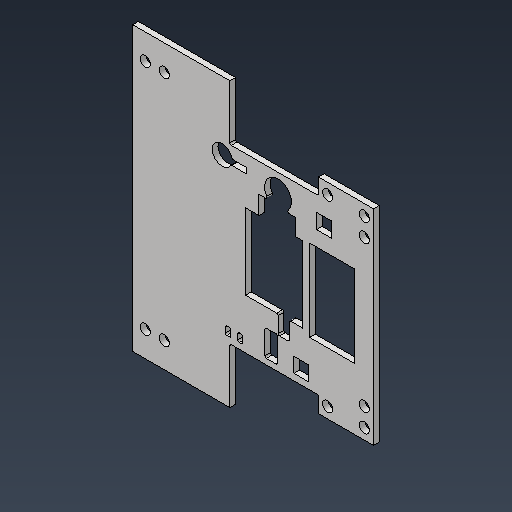
# Autodesk Inventor part: ceil
Saved by Autodesk Inventor 2026.2 (Build 302298010, 298A)
## iProperties
Created: 2026-05-09
Part Number: ceil
Material: Generic
Document SubType Name: Modeling
Designer: szymo
Density: 1 g/cm^3
Appearance: Default
Author: szymo
Autodesk Inventor part; units mm, degrees
ref_plane "YZ Plane" through (0, 0, 0) normal (1, 0, 0) x (0, 1, 0)
ref_plane "XZ Plane" through (0, 0, 0) normal (0, 1, 0) x (-1, 0, 0)
ref_plane "XY Plane" through (0, 0, 0) normal (0, 0, 1) x (1, 0, 0)
sketch "Sketch1" plane through (0, 0, 0) normal (0, 0, 1) x (1, 0, 0)
  circle A0 centre (3.25, 13.15) radius 1.2295 projected
  line L0 (0, 9.3) -> (6.5, 9.3) projected
  line L1 (6.5, 9.3) -> (6.5, 17) projected
  line L2 (0, 17) -> (6.5, 17) projected
  line L3 (0, 9.3) -> (0, 17) projected
  circle A1 centre (3.25, 6.65) radius 1.2295 projected
  line L4 (0, 0) -> (6.5, 0) projected
  line L5 (6.5, 0) -> (6.5, 9.3) projected
  line L6 (6.5, 9.3) -> (0, 9.3) projected
  line L7 (0, 0) -> (0, 9.3) projected
  circle A2 centre (-9.75, 13.15) radius 1.2295 projected
  line L8 (-41.3371, 11.3) -> (-13, 11.3) projected
  line L9 (-41.3371, 9.3) -> (-41.3371, 11.3) projected
  line L10 (-41.3371, 9.3) -> (-6.5, 9.3) projected
  line L11 (-6.5, 9.3) -> (-6.5, 17) projected
  line L12 (-13, 17) -> (-6.5, 17) projected
  line L13 (-13, 11.3) -> (-13, 17) projected
  circle A3 centre (3.25, -51.55) radius 1.2295 projected
  line L14 (0, -47.7) -> (6.5, -47.7) projected
  line L15 (0, -47.7) -> (0, -55.4) projected
  line L16 (6.5, -55.4) -> (0, -55.4) projected
  line L17 (6.5, -47.7) -> (6.5, -55.4) projected
  circle A4 centre (3.25, -45.05) radius 1.2295 projected
  line L18 (0.5983, -42.4) -> (0, -42.4) projected
  line L19 (0, -42.4) -> (0, -47.7) projected
  line L20 (0, -47.7) -> (6.5, -47.7) projected
  line L21 (6.5, -38.4) -> (6.5, -47.7) projected
  line L22 (0.5983, -38.4) -> (6.5, -38.4) projected
  line L23 (0.5983, -38.4) -> (0.5983, -42.4) projected
  circle A5 centre (-9.75, -51.55) radius 1.2295 projected
  line L24 (-41.3371, -47.7) -> (-6.5, -47.7) projected
  line L25 (-41.3371, -47.7) -> (-41.3371, -49.7) projected
  line L26 (-13, -49.7) -> (-41.3371, -49.7) projected
  line L27 (-13, -49.7) -> (-13, -55.4) projected
  line L28 (-6.5, -55.4) -> (-13, -55.4) projected
  line L29 (-6.5, -47.7) -> (-6.5, -55.4) projected
  circle A6 centre (-67.4121, -60.2) radius 1.2295 projected
  circle A7 centre (-74.1621, -60.2) radius 1.2295 projected
  arc A8 (-64.1621, -55.1072) -> (-64.7971, -54.6257) centre (-64.6621, -55.1072) ccw projected
  arc A9 (-65.3371, -54.7) -> (-64.7971, -54.6257) centre (-65.3371, -52.7) ccw projected
  line L30 (-65.3371, -54.7) -> (-78.8451, -54.7) projected
  line L31 (-78.8451, -54.7) -> (-78.8451, -69.2) projected
  line L32 (-59.3371, -69.2) -> (-78.8451, -69.2) projected
  line L33 (-59.3371, -67.7) -> (-59.3371, -69.2) projected
  line L34 (-59.3371, -67.7) -> (-70.1621, -67.7) projected
  line L35 (-70.1621, -67.7) -> (-70.1621, -65.2) projected
  line L36 (-70.1621, -65.2) -> (-67.1621, -65.2) projected
  arc A10 (-67.1621, -65.2) -> (-64.1621, -62.2) centre (-67.1621, -62.2) ccw projected
  line L37 (-64.1621, -62.2) -> (-64.1621, -55.1072) projected
  arc A11 (-64.7971, 16.2257) -> (-64.1621, 16.7072) centre (-64.6621, 16.7072) ccw projected
  line L38 (-64.1621, 16.7072) -> (-64.1621, 23.8) projected
  arc A12 (-64.1621, 23.8) -> (-67.1621, 26.8) centre (-67.1621, 23.8) ccw projected
  line L39 (-67.1621, 26.8) -> (-70.1621, 26.8) projected
  line L40 (-70.1621, 26.8) -> (-70.1621, 29.3) projected
  line L41 (-70.1621, 29.3) -> (-59.3371, 29.3) projected
  line L42 (-59.3371, 29.3) -> (-59.3371, 30.8) projected
  line L43 (-59.3371, 30.8) -> (-78.8451, 30.8) projected
  line L44 (-78.8451, 16.3) -> (-78.8451, 30.8) projected
  line L45 (-65.3371, 16.3) -> (-78.8451, 16.3) projected
  arc A13 (-64.7971, 16.2257) -> (-65.3371, 16.3) centre (-65.3371, 14.3) ccw projected
  circle A14 centre (-67.4121, 21.8) radius 1.2295 projected
  circle A15 centre (-74.1621, 21.8) radius 1.2295 projected
  line L46 (-78.5805, 30.8) -> (-78.5805, -69.2) projected
  line L47 (-44.2868, 25.8) -> (-44.2868, 15.8) projected
  line L48 (-44.2868, -54.2) -> (-44.2868, -64.2) projected
  line L49 (-59.3371, 30.8) -> (-44.2868, 30.8)
  line L50 (-44.2868, 30.8) -> (-44.2868, 11.3)
  line L51 (-44.2868, 11.3) -> (-41.3371, 11.3)
  line L52 (-59.3371, -69.2) -> (-44.2868, -69.2)
  line L53 (-44.2868, -69.2) -> (-44.2868, -64.2)
  line L54 (-44.2868, -54.2) -> (-44.2868, -49.7)
  line L55 (-44.2868, -49.7) -> (-41.3371, -49.7)
  line L56 (-6.5, 17) -> (0, 17)
  line L57 (6.5, 0) -> (6.5, -38.4)
  line L58 (0, -55.4) -> (-6.5, -55.4)
  line L59 (-24.2185, -0.425) -> (-24.4685, -0.675) construction
  line L60 (-24.4685, -0.675) -> (-24.4685, -0.725) construction
  line L61 (-24.4685, -0.725) -> (-24.5685, -0.725) construction
  line L62 (-24.5685, -5.125) -> (-24.5685, -0.725) construction
  line L63 (-24.4685, -5.125) -> (-24.5685, -5.125) construction
  line L64 (-24.4685, -5.125) -> (-24.4685, -5.175) construction
  line L65 (-24.4685, -5.175) -> (-24.2185, -5.425) construction
  line L66 (-24.2185, -5.425) -> (-23.3685, -5.425) construction
  line L67 (-23.3685, -5.925) -> (-23.3685, -5.425) construction
  line L68 (-21.6685, -5.925) -> (-23.3685, -5.925) construction
  line L69 (-21.6685, -5.925) -> (-21.6685, 0.075) construction
  line L70 (-21.6685, 0.075) -> (-23.3685, 0.075) construction
  line L71 (-23.3685, 0.075) -> (-23.3685, -0.425) construction
  line L72 (-24.2185, -0.425) -> (-23.3685, -0.425) construction
  line L73 (-24.2685, -5.225) -> (-23.1685, -5.225) construction
  line L74 (-24.2685, -0.625) -> (-24.2685, -5.225) construction
  line L75 (-24.2685, -0.625) -> (-23.1685, -0.625) construction
  line L76 (-23.1685, -0.625) -> (-23.1685, -0.375) construction
  line L77 (-22.5685, -0.375) -> (-23.1685, -0.375) construction
  line L78 (-22.5685, -0.375) -> (-22.5685, -0.625) construction
  line L79 (-22.5685, -0.625) -> (-21.9685, -0.625) construction
  line L80 (-21.9685, -5.225) -> (-21.9685, -0.625) construction
  line L81 (-22.5685, -5.225) -> (-21.9685, -5.225) construction
  line L82 (-22.5685, -5.475) -> (-22.5685, -5.225) construction
  line L83 (-22.5685, -5.475) -> (-23.1685, -5.475) construction
  line L84 (-23.1685, -5.225) -> (-23.1685, -5.475) construction
  line L85 (-30.9685, -4.8) -> (-30.7185, -4.55) construction
  line L86 (-30.7185, -4.55) -> (-30.7185, -4.5) construction
  line L87 (-30.7185, -4.5) -> (-30.6185, -4.5) construction
  line L88 (-30.6185, -0.1) -> (-30.6185, -4.5) construction
  line L89 (-30.7185, -0.1) -> (-30.6185, -0.1) construction
  line L90 (-30.7185, -0.1) -> (-30.7185, -0.05) construction
  line L91 (-30.7185, -0.05) -> (-30.9685, 0.2) construction
  line L92 (-30.9685, 0.2) -> (-31.8185, 0.2) construction
  line L93 (-31.8185, 0.7) -> (-31.8185, 0.2) construction
  line L94 (-33.5185, 0.7) -> (-31.8185, 0.7) projected
  line L95 (-33.5185, 0.7) -> (-33.5185, -5.3) construction
  line L96 (-33.5185, -5.3) -> (-31.8185, -5.3) construction
  line L97 (-31.8185, -5.3) -> (-31.8185, -4.8) construction
  line L98 (-30.9685, -4.8) -> (-31.8185, -4.8) construction
  line L99 (-30.9185, 0) -> (-32.0185, 0) construction
  line L100 (-30.9185, -4.6) -> (-30.9185, 0) construction
  line L101 (-30.9185, -4.6) -> (-32.0185, -4.6) construction
  line L102 (-32.0185, -4.6) -> (-32.0185, -4.85) construction
  line L103 (-32.6185, -4.85) -> (-32.0185, -4.85) construction
  line L104 (-32.6185, -4.85) -> (-32.6185, -4.6) construction
  line L105 (-32.6185, -4.6) -> (-33.2185, -4.6) construction
  line L106 (-33.2185, 0) -> (-33.2185, -4.6) construction
  line L107 (-32.6185, 0) -> (-33.2185, 0) construction
  line L108 (-32.6185, 0.25) -> (-32.6185, 0) construction
  line L109 (-32.6185, 0.25) -> (-32.0185, 0.25) construction
  line L110 (-32.0185, 0) -> (-32.0185, 0.25) construction
  line L111 (-26.3685, -32.525) -> (-26.6185, -32.775) construction
  line L112 (-26.6185, -32.775) -> (-26.6185, -32.825) construction
  line L113 (-26.6185, -32.825) -> (-26.7185, -32.825) construction
  line L114 (-26.7185, -37.225) -> (-26.7185, -32.825) construction
  line L115 (-26.6185, -37.225) -> (-26.7185, -37.225) construction
  line L116 (-26.6185, -37.225) -> (-26.6185, -37.275) construction
  line L117 (-26.6185, -37.275) -> (-26.3685, -37.525) construction
  line L118 (-26.3685, -37.525) -> (-25.5185, -37.525) construction
  line L119 (-25.5185, -38.025) -> (-25.5185, -37.525) construction
  line L120 (-23.8185, -38.025) -> (-25.5185, -38.025) construction
  line L121 (-23.8185, -38.025) -> (-23.8185, -32.025) construction
  line L122 (-23.8185, -32.025) -> (-25.5185, -32.025) construction
  line L123 (-25.5185, -32.025) -> (-25.5185, -32.525) construction
  line L124 (-26.3685, -32.525) -> (-25.5185, -32.525) construction
  line L125 (-26.4185, -37.325) -> (-25.3185, -37.325) construction
  line L126 (-26.4185, -32.725) -> (-26.4185, -37.325) construction
  line L127 (-26.4185, -32.725) -> (-25.3185, -32.725) construction
  line L128 (-25.3185, -32.725) -> (-25.3185, -32.475) construction
  line L129 (-24.7185, -32.475) -> (-25.3185, -32.475) construction
  line L130 (-24.7185, -32.475) -> (-24.7185, -32.725) construction
  line L131 (-24.7185, -32.725) -> (-24.1185, -32.725) construction
  line L132 (-24.1185, -37.325) -> (-24.1185, -32.725) construction
  line L133 (-24.7185, -37.325) -> (-24.1185, -37.325) construction
  line L134 (-24.7185, -37.575) -> (-24.7185, -37.325) construction
  line L135 (-24.7185, -37.575) -> (-25.3185, -37.575) construction
  line L136 (-25.3185, -37.325) -> (-25.3185, -37.575) construction
  line L137 (-28.2435, -45.725) -> (-28.2435, -46.975) construction
  line L138 (-27.8935, -45.725) -> (-28.2435, -45.725) construction
  line L139 (-27.8935, -40.225) -> (-27.8935, -45.725) construction
  line L140 (-27.8935, -40.225) -> (-28.2435, -40.225) construction
  line L141 (-28.2435, -40.225) -> (-28.2435, -38.975) construction
  line L142 (-28.7927, -38.975) -> (-28.2435, -38.975) construction
  line L143 (-28.7927, -38.975) -> (-30.4943, -38.975) construction
  line L144 (-30.4943, -38.975) -> (-31.0435, -38.975) construction
  line L145 (-31.0435, -40.225) -> (-31.0435, -38.975) construction
  line L146 (-31.3935, -40.225) -> (-31.0435, -40.225) construction
  line L147 (-31.3935, -40.225) -> (-31.3935, -45.725) construction
  line L148 (-31.3935, -45.725) -> (-31.0435, -45.725) construction
  line L149 (-31.0435, -45.725) -> (-31.0435, -46.975) construction
  line L150 (-30.4943, -46.975) -> (-31.0435, -46.975) construction
  line L151 (-28.7927, -46.975) -> (-30.4943, -46.975) construction
  line L152 (-28.7927, -46.975) -> (-28.2435, -46.975) construction
  line L153 (-30.7273, -45.075) -> (-30.7273, -40.875) construction
  line L154 (-30.7273, -40.875) -> (-28.5597, -40.875) construction
  line L155 (-28.5597, -45.075) -> (-28.5597, -40.875) construction
  line L156 (-30.7273, -45.075) -> (-28.5597, -45.075) construction
  line L157 (-41.0185, -45.5213) -> (-41.0185, -46.4787) projected
  line L158 (-40.3185, -46.4787) -> (-41.0185, -46.4787) projected
  line L159 (-40.3185, -45.5213) -> (-40.3185, -46.4787) projected
  line L160 (-40.3185, -45.5213) -> (-41.0185, -45.5213) projected
  line L161 (-45.335, -45.95) -> (-44.3776, -45.95) projected
  line L162 (-44.3776, -45.25) -> (-44.3776, -45.95) projected
  line L163 (-45.335, -45.25) -> (-44.3776, -45.25) projected
  line L164 (-45.335, -45.25) -> (-45.335, -45.95) projected
  line L165 (-45.335, -47.15) -> (-44.3776, -47.15) projected
  line L166 (-44.3776, -46.45) -> (-44.3776, -47.15) projected
  line L167 (-45.335, -46.45) -> (-44.3776, -46.45) projected
  line L168 (-45.335, -46.45) -> (-45.335, -47.15) projected
  line L169 (-17.9153, -43.2723) -> (-20.1185, -43.2723) construction
  line L170 (-20.1185, -43.2723) -> (-20.1185, -46.3457) construction
  line L171 (-20.1185, -46.3457) -> (-17.9153, -46.3457) construction
  line L172 (-17.9153, -46.3457) -> (-17.9153, -43.2723) construction
  circle A16 centre (-19.0169, -44.809) radius 0.1905 construction
  line L173 (-19.3137, -44.1058) -> (-19.7201, -44.1058) construction
  line L174 (-19.3137, -44.5122) -> (-19.3137, -44.1058) construction
  line L175 (-19.7201, -44.5122) -> (-19.3137, -44.5122) construction
  line L176 (-19.7201, -44.1058) -> (-19.7201, -44.5122) construction
  line L177 (-19.3137, -45.1058) -> (-19.7201, -45.1058) construction
  line L178 (-19.3137, -45.5122) -> (-19.3137, -45.1058) construction
  line L179 (-19.7201, -45.5122) -> (-19.3137, -45.5122) construction
  line L180 (-19.7201, -45.1058) -> (-19.7201, -45.5122) construction
  line L181 (-18.3137, -44.1058) -> (-18.7201, -44.1058) construction
  line L182 (-18.3137, -44.5122) -> (-18.3137, -44.1058) construction
  line L183 (-18.7201, -44.5122) -> (-18.3137, -44.5122) construction
  line L184 (-18.7201, -44.1058) -> (-18.7201, -44.5122) construction
  line L185 (-18.3137, -45.1058) -> (-18.7201, -45.1058) construction
  line L186 (-18.3137, -45.5122) -> (-18.3137, -45.1058) construction
  line L187 (-18.7201, -45.5122) -> (-18.3137, -45.5122) construction
  line L188 (-18.7201, -45.1058) -> (-18.7201, -45.5122) construction
  line L189 (-12.1467, 1.6723) -> (-9.9435, 1.6723) construction
  line L190 (-9.9435, 1.6723) -> (-9.9435, 4.7457) construction
  line L191 (-9.9435, 4.7457) -> (-12.1467, 4.7457) construction
  line L192 (-12.1467, 4.7457) -> (-12.1467, 1.6723) construction
  circle A17 centre (-11.0451, 3.209) radius 0.1905 construction
  line L193 (-10.7483, 2.5058) -> (-10.3419, 2.5058) construction
  line L194 (-10.7483, 2.9122) -> (-10.7483, 2.5058) construction
  line L195 (-10.3419, 2.9122) -> (-10.7483, 2.9122) construction
  line L196 (-10.3419, 2.5058) -> (-10.3419, 2.9122) construction
  line L197 (-10.7483, 3.5058) -> (-10.3419, 3.5058) construction
  line L198 (-10.7483, 3.9122) -> (-10.7483, 3.5058) construction
  line L199 (-10.3419, 3.9122) -> (-10.7483, 3.9122) construction
  line L200 (-10.3419, 3.5058) -> (-10.3419, 3.9122) construction
  line L201 (-11.7483, 2.5058) -> (-11.3419, 2.5058) construction
  line L202 (-11.7483, 2.9122) -> (-11.7483, 2.5058) construction
  line L203 (-11.3419, 2.9122) -> (-11.7483, 2.9122) construction
  line L204 (-11.3419, 2.5058) -> (-11.3419, 2.9122) construction
  line L205 (-11.7483, 3.5058) -> (-11.3419, 3.5058) construction
  line L206 (-11.7483, 3.9122) -> (-11.7483, 3.5058) construction
  line L207 (-11.3419, 3.9122) -> (-11.7483, 3.9122) construction
  line L208 (-11.3419, 3.5058) -> (-11.3419, 3.9122) construction
  line L209 (-23.8672, 6.1175) -> (-23.9186, 6.0661) projected
  line L210 (-23.9186, 6.0661) -> (-24.3824, 6.53) projected
  line L211 (-24.3824, 6.53) -> (-25.2253, 6.595) projected
  line L212 (-25.2969, 7.4444) -> (-25.2253, 6.595) projected
  line L213 (-25.2969, 7.4444) -> (-25.7614, 7.9089) projected
  line L214 (-25.71, 7.9603) -> (-25.7614, 7.9089) projected
  line L215 (-25.71, 7.9603) -> (-26.2969, 8.5472) projected
  line L216 (-26.2969, 8.5472) -> (-26.3131, 8.5309) projected
  line L217 (-26.3131, 8.5309) -> (-26.5472, 8.765) projected
  arc A18 (-26.5721, 8.7467) -> (-26.5472, 8.765) centre (-26.6195, 8.8373) ccw projected
  line L218 (-26.5721, 8.7467) -> (-28.0279, 8.7049) projected
  line L219 (-28.0279, 8.7049) -> (-31.3307, 5.4022) projected
  arc A19 (-31.3399, 5.3203) -> (-31.3307, 5.4022) centre (-31.5512, 5.3856) ccw projected
  line L220 (-31.4669, 3.8791) -> (-31.3399, 5.3203) projected
  arc A20 (-31.4965, 3.8157) -> (-31.4669, 3.8791) centre (-31.5688, 3.888) ccw projected
  line L221 (-31.2624, 3.5817) -> (-31.4965, 3.8157) projected
  line L222 (-31.2787, 3.5654) -> (-31.2624, 3.5817) projected
  line L223 (-31.2787, 3.5654) -> (-30.6918, 2.9785) projected
  line L224 (-30.6918, 2.9785) -> (-30.6404, 3.0299) projected
  line L225 (-28.7976, 1.1871) -> (-30.6404, 3.0299) projected
  line L226 (-28.849, 1.1357) -> (-28.7976, 1.1871) projected
  line L227 (-28.849, 1.1357) -> (-28.2621, 0.5488) projected
  line L228 (-28.2621, 0.5488) -> (-28.2458, 0.5651) projected
  line L229 (-28.2458, 0.5651) -> (-27.9616, 0.2808) projected
  arc A21 (-27.893, 0.3051) -> (-27.9616, 0.2808) centre (-27.9018, 0.2211) ccw projected
  line L230 (-27.893, 0.3051) -> (-26.5072, 0.4876) projected
  arc A22 (-26.4091, 0.495) -> (-26.5072, 0.4876) centre (-26.4419, 0.2763) ccw projected
  line L231 (-26.4091, 0.495) -> (-23.1694, 3.7347) projected
  line L232 (-23.092, 5.2169) -> (-23.1694, 3.7347) projected
  arc A23 (-23.0625, 5.2802) -> (-23.092, 5.2169) centre (-22.9902, 5.208) ccw projected
  line L233 (-23.2966, 5.5143) -> (-23.0625, 5.2802) projected
  line L234 (-23.2803, 5.5306) -> (-23.2966, 5.5143) projected
  line L235 (-23.2803, 5.5306) -> (-23.8672, 6.1175) projected
  line L236 (-39.4685, 6.6787) -> (-39.4685, 5.7213) projected
  line L237 (-38.7685, 5.7213) -> (-39.4685, 5.7213) projected
  line L238 (-38.7685, 6.6787) -> (-38.7685, 5.7213) projected
  line L239 (-38.7685, 6.6787) -> (-39.4685, 6.6787) projected
  line L240 (-41.6435, 6.7037) -> (-41.6435, 5.7463) projected
  line L241 (-40.9435, 5.7463) -> (-41.6435, 5.7463) projected
  line L242 (-40.9435, 6.7037) -> (-40.9435, 5.7463) projected
  line L243 (-40.9435, 6.7037) -> (-41.6435, 6.7037) projected
  line L244 (-43.8685, 6.6659) -> (-43.8685, 5.7085) construction
  line L245 (-43.1685, 5.7085) -> (-43.8685, 5.7085) construction
  line L246 (-43.1685, 6.6659) -> (-43.1685, 5.7085) projected
  line L247 (-43.1685, 6.6659) -> (-43.8685, 6.6659) construction
  line L248 (-48.9685, 4.8) -> (-48.9685, 8.75) construction
  line L249 (-45.0185, 4.8) -> (-48.9685, 4.8) construction
  line L250 (-45.0185, 8.75) -> (-45.0185, 4.8) construction
  line L251 (-48.9685, 8.75) -> (-45.0185, 8.75) construction
  line L252 (-8.4451, 0.559) -> (-13.6451, 0.559)
  line L253 (-13.6451, 0.559) -> (-13.6451, 5.859)
  line L254 (-13.6451, 5.859) -> (-8.4451, 5.859)
  line L255 (-8.4451, 5.859) -> (-8.4451, 0.559)
  line L256 (-8.4451, 0.559) -> (-13.6451, 5.859) construction
  line L257 (-13.6451, 0.559) -> (-8.4451, 5.859) construction
  line L258 (-21.6169, -42.209) -> (-16.4169, -42.209)
  line L259 (-16.4169, -42.209) -> (-16.4169, -47.409)
  line L260 (-16.4169, -47.409) -> (-21.6169, -47.409)
  line L261 (-21.6169, -47.409) -> (-21.6169, -42.209)
  line L262 (-21.6169, -42.209) -> (-16.4169, -47.409) construction
  line L263 (-16.4169, -42.209) -> (-21.6169, -47.409) construction
  line L264 (-0.7973, -5.25) -> (-0.7973, -33.15)
  line L265 (-0.7973, -33.15) -> (-2.3085, -33.15)
  line L266 (-2.3085, -33.15) -> (-2.3085, -5.25)
  line L267 (-2.3085, -5.25) -> (-0.7973, -5.25)
  line L268 (-15.6027, -33.15) -> (-15.6027, -5.25)
  line L269 (-15.6027, -5.25) -> (-14.0915, -5.25)
  line L270 (-14.0915, -5.25) -> (-14.0915, -33.15)
  line L271 (-14.0915, -33.15) -> (-15.6027, -33.15)
  line L272 (-41.7344, -5.25) -> (-41.7344, -33.15)
  line L273 (-41.7344, -33.15) -> (-43.2456, -33.15)
  line L274 (-43.2456, -33.15) -> (-43.2456, -5.25)
  line L275 (-43.2456, -5.25) -> (-41.7344, -5.25)
  line L276 (-56.5398, -33.15) -> (-56.5398, -5.25)
  line L277 (-56.5398, -5.25) -> (-55.0286, -5.25)
  line L278 (-55.0286, -5.25) -> (-55.0286, -33.15)
  line L279 (-55.0286, -33.15) -> (-56.5398, -33.15)
  line L280 (-18.6027, -5.3) -> (-38.7344, -5.3)
  line L281 (-38.7344, -5.3) -> (-38.7344, -32.025)
  line L282 (-38.7344, -32.025) -> (-18.6027, -32.025)
  line L283 (-18.6027, -32.025) -> (-18.6027, -5.3)
  line L284 (-41.2344, -4.75) -> (-57.0398, -4.75)
  line L285 (-57.0398, -4.75) -> (-57.0398, -33.65)
  line L286 (-57.0398, -33.65) -> (-41.2344, -33.65)
  line L287 (-41.2344, -33.65) -> (-41.2344, -4.75)
  line L288 (-16.1027, -4.75) -> (-0.2973, -4.75)
  line L289 (-0.2973, -4.75) -> (-0.2973, -33.65)
  line L290 (-0.2973, -33.65) -> (-16.1027, -33.65)
  line L291 (-16.1027, -33.65) -> (-16.1027, -4.75)
  circle A24 centre (-27.275, 4.5435) radius 1.5 projected
  circle A25 centre (-27.275, 4.5435) radius 4.7565
  line L292 (-45.0185, 8.75) -> (-48.9685, 4.8) construction
  line L293 (-48.9685, 8.75) -> (-45.0185, 4.8) construction
  circle A26 centre (-46.9935, 6.775) radius 3.5
  line L294 (-38.2685, 7.2037) -> (-44.3685, 7.2037)
  line L295 (-44.3685, 7.2037) -> (-44.3685, 5.2463)
  line L296 (-44.3685, 5.2463) -> (-38.2685, 5.2463)
  line L297 (-38.2685, 5.2463) -> (-38.2685, 7.2037)
  line L298 (-39.8185, -47.65) -> (-45.835, -47.65)
  line L299 (-45.835, -47.65) -> (-45.835, -44.75)
  line L300 (-45.835, -44.75) -> (-39.8185, -44.75)
  line L301 (-39.8185, -44.75) -> (-39.8185, -47.65)
  line L302 (-27.2185, -38.525) -> (-23.3185, -38.525)
  line L303 (-23.3185, -38.525) -> (-23.3185, -31.525)
  line L304 (-23.3185, -31.525) -> (-27.2185, -31.525)
  line L305 (-27.2185, -31.525) -> (-27.2185, -38.525)
  line L306 (-31.8935, -38.475) -> (-27.3935, -38.475)
  line L307 (-27.3935, -38.475) -> (-27.3935, -47.7)
  line L308 (-27.3935, -47.7) -> (-31.8935, -47.7)
  line L309 (-31.8935, -47.7) -> (-31.8935, -38.475)
  line L310 (-21.1685, 0.575) -> (-25.0685, 0.575)
  line L311 (-25.0685, 0.575) -> (-25.0685, -6.425)
  line L312 (-25.0685, -6.425) -> (-21.1685, -6.425)
  line L313 (-21.1685, -6.425) -> (-21.1685, 0.575)
  line L314 (-34.0185, -5.8) -> (-30.1185, -5.8)
  line L315 (-30.1185, -5.8) -> (-30.1185, 1.2)
  line L316 (-30.1185, 1.2) -> (-34.0185, 1.2)
  line L317 (-34.0185, 1.2) -> (-34.0185, -5.8)
  line L318 (-41.5185, -44.75) -> (-43.8776, -44.75)
  line L319 (-43.8776, -44.75) -> (-43.8776, -47.65)
  line L320 (-43.8776, -47.65) -> (-41.5185, -47.65)
  line L321 (-41.5185, -47.65) -> (-41.5185, -44.75)
  point P0 (-55.5286, -5.25)
  point P1 (-55.5286, -33.15)
  point P2 (-24.6529, 0.575)
  point P3 (-25.0685, 0.3298)
  point P4 (-30.1185, 0.7305)
  point P5 (-30.6581, 1.2)
  point P6 (-43.845, 5.2463)
  point P7 (-43.5199, 7.2037)
  point P8 (-21.1685, -5.3)
  point P9 (-23.3185, -32.025)
  point P10 (-27.2185, -32.025)
  point P11 (-34.0185, -5.3)
  dimension "d2" = 5.2
  dimension "d3" = 5.3
  dimension "d4" = 5.2
  dimension "d5" = 5.2
  dimension "d7" = 0
  dimension "d8" = 3
  dimension "d9" = 3
  dimension "d11" = 0.5
  dimension "d12" = 0.5
  dimension "d13" = 0.5
  dimension "d14" = 0.5
  dimension "d15" = 0.5
  dimension "d16" = 0.5
  dimension "d17" = 0.5
  dimension "d18" = 0.5
  dimension "d19" = 7
  dimension "d20" = 0.5
  dimension "d21" = 0.5
  dimension "d22" = 0.5
  dimension "d23" = 0.5
  dimension "d25" = 0.5
  dimension "d27" = 0.5
  dimension "d28" = 0.5
  dimension "d29" = 0.5
  dimension "d30" = 0.5
  dimension "d31" = 0.5
  dimension "d32" = 0.5
  dimension "d33" = 0.5
  dimension "d34" = 0.5
  dimension "d35" = 0.5
  dimension "d36" = 0.5
  dimension "d37" = 0.5
  dimension "d38" = 0.5
  dimension "d39" = 0.5
  dimension "d40" = 0.5
  dimension "d41" = 0.5
  dimension "d42" = 0.5
  dimension "d43" = 0.5
  dimension "d44" = 0.5
  dimension "d45" = 0.5
  dimension "d46" = 0.5
  dimension "d55" = 0
  constraints: 160 end point, 25 parallel, 21 horizontal, 16 perpendicular, 9 vertical, 5 midpoint, 5 point on line, 2 centre point, 1 coincident, 1 collinear, 1 tangent, 16 other
  measures "d2" distance of L253.end L254.end
  measures "d3" distance of L252.end L253.end
  measures "d4" distance of L259.end L260.end
  measures "d5" distance of L258.end L259.end
  measures "d7" distance from line of L121.end L282
  measures "d8" distance between parallel lines of L268 L283
  measures "d9" distance between parallel lines of L272 L281
  measures "d11" distance between parallel lines of L284 L277
  measures "d12" distance between parallel lines of L286 L279
  measures "d13" distance between parallel lines of L287 L272
  measures "d14" distance between parallel lines of L291 L268
  measures "d15" distance between parallel lines of L288 L269
  measures "d16" distance between parallel lines of L271 L290
  measures "d17" distance between parallel lines of L289 L264
  measures "d18" distance between parallel lines of L285 L276
  measures "d19" diameter of A26
  measures "d20" distance from line of L296 L241.start
  measures "d21" distance from line of L294 L242.start
  measures "d22" distance from line of L297 L238.start
  measures "d23" distance from line of L295 L244.start
  measures "d25" distance from line of L301 L158.start
  measures "d27" distance from line of L299 L163.start
  measures "d28" distance from line of L298 L165.start
  measures "d29" distance from line of L300 L163.start
  measures "d30" distance from line of L307 L138.start
  measures "d31" distance from line of L306 L141.end
  measures "d32" distance from line of L309 L146.start
  measures "d33" distance from line of L114.start L305
  measures "d34" distance from line of L302 L120.start
  measures "d35" distance from line of L303 L121.end
  measures "d36" distance from line of L304 L121.end
  measures "d37" distance from line of L310 L69.end
  measures "d38" distance from line of L313 L68.start
  measures "d39" distance from line of L311 L62.start
  measures "d40" distance from line of L67.start L312
  measures "d41" distance from line of L315 L88.start
  measures "d42" distance from line of L316 L94.start
  measures "d43" distance from line of L94.start L317
  measures "d44" distance from line of L314 L95.end
  measures "d45" distance from line of L161.end L319
  measures "d46" distance from line of L157.end L321
  measures "d55" distance from line of L280 L96.end
extrude "Extrusion1" add sketch "Sketch1" along normal blind 2 contours A0 | L3 L2 L1 L0 | L7 L4 L57 L22 L23 L18 L19 L15 L58 L29 L24 L307 L306 L309 L25 L55 L54 L48 L53 L52 L33 L34 L35 L36 A10 L37 A8 A9 L30 L46 L45 A13 A11 L38 A12 L39 L40 L41 L42 L49 L50 L47 L51 L9 L10 L11 L56 L3 | L0 L5 L4 L7 | L11 L10 L9 L8 L13 L12 | L21 L14 L19 L18 L23 L22 | L17 L16 L15 L14 | L28 L27 L26 L25 L24 L29 | L42 L41 L40 L39 A12 L38 A11 A13 L45 L46 L43 | L30 A9 A8 L37 A10 L36 L35 L34 L33 L32 L46 | A1 | A2 | A3 | A4 | A5 | A6 | A7 | A14 | A15 | L272 L273 L274 L275 | L276 L277 L278 L279 | L287 L286 L285 L284 | L298 L319 L300 L321
fillet "Fillet1" radius 0.5 27 edges at (-24.6529, 0.575, 1) (-30.6581, 1.2, 1) (-43.845, 5.2463, 1) (-43.5199, 7.2037, 1) (-38.2685, 7.2037, 1) (-38.2685, 5.2463, 1) (-45.835, -47.65, 1) (-45.835, -44.75, 1) (-43.8776, -44.75, 1) (-43.8776, -47.65, 1) (-41.5185, -47.65, 1) (-41.5185, -44.75, 1) (-39.8185, -44.75, 1) (-39.8185, -47.65, 1) (-27.3935, -47.7, 1) (-31.8935, -47.7, 1) (-31.8935, -38.475, 1) (-27.3935, -38.475, 1) (-27.2185, -38.525, 1) (-23.3185, -38.525, 1) (-23.3185, -32.025, 1) (-27.2185, -32.025, 1) (-21.1685, -5.3, 1) (-13, 11.3, 1) (-44.2868, 11.3, 1) (-44.2868, -49.7, 1) (-13, -49.7, 1)
sketch "Sketch2" plane through (0, 0, 2) normal (0, 0, 1) x (1, 0, 0)
  circle A0 centre (3.25, 13.15) radius 1.2295 projected
  line L0 (0, 9.3) -> (6.5, 9.3) projected
  line L1 (6.5, 9.3) -> (6.5, 17) projected
  line L2 (0, 17) -> (6.5, 17) projected
  line L3 (0, 9.3) -> (0, 17) projected
  circle A1 centre (3.25, 6.65) radius 1.2295 projected
  line L4 (0, 0) -> (6.5, 0) projected
  line L5 (6.5, 0) -> (6.5, 9.3) projected
  line L6 (6.5, 9.3) -> (0, 9.3) projected
  line L7 (0, 0) -> (0, 9.3) projected
  circle A2 centre (-9.75, 13.15) radius 1.2295 projected
  line L8 (-41.3371, 11.3) -> (-13, 11.3) projected
  line L9 (-41.3371, 9.3) -> (-41.3371, 11.3) projected
  line L10 (-41.3371, 9.3) -> (-6.5, 9.3) projected
  line L11 (-6.5, 9.3) -> (-6.5, 17) projected
  line L12 (-13, 17) -> (-6.5, 17) projected
  line L13 (-13, 11.3) -> (-13, 17) projected
  circle A3 centre (3.25, -51.55) radius 1.2295 projected
  line L14 (0, -47.7) -> (6.5, -47.7) projected
  line L15 (0, -47.7) -> (0, -55.4) projected
  line L16 (6.5, -55.4) -> (0, -55.4) projected
  line L17 (6.5, -47.7) -> (6.5, -55.4) projected
  circle A4 centre (3.25, -45.05) radius 1.2295 projected
  line L18 (0.5983, -42.4) -> (0, -42.4) projected
  line L19 (0, -42.4) -> (0, -47.7) projected
  line L20 (0, -47.7) -> (6.5, -47.7) projected
  line L21 (6.5, -38.4) -> (6.5, -47.7) projected
  line L22 (0.5983, -38.4) -> (6.5, -38.4) projected
  line L23 (0.5983, -38.4) -> (0.5983, -42.4) projected
  circle A5 centre (-9.75, -51.55) radius 1.2295 projected
  line L24 (-41.3371, -47.7) -> (-6.5, -47.7) projected
  line L25 (-41.3371, -47.7) -> (-41.3371, -49.7) projected
  line L26 (-13, -49.7) -> (-41.3371, -49.7) projected
  line L27 (-13, -49.7) -> (-13, -55.4) projected
  line L28 (-6.5, -55.4) -> (-13, -55.4) projected
  line L29 (-6.5, -47.7) -> (-6.5, -55.4) projected
  line L30 (-61.1621, -61.725) -> (-76.1621, -61.725) projected
  circle A6 centre (-67.4121, -60.2) radius 1.2295 projected
  circle A7 centre (-74.1621, -60.2) radius 1.2295 projected
  arc A8 (-64.1621, -55.1072) -> (-64.7971, -54.6257) centre (-64.6621, -55.1072) ccw projected
  arc A9 (-65.3371, -54.7) -> (-64.7971, -54.6257) centre (-65.3371, -52.7) ccw projected
  line L31 (-65.3371, -54.7) -> (-78.8451, -54.7) projected
  line L32 (-78.8451, -54.7) -> (-78.8451, -69.2) projected
  line L33 (-59.3371, -69.2) -> (-78.8451, -69.2) projected
  line L34 (-59.3371, -67.7) -> (-59.3371, -69.2) projected
  line L35 (-59.3371, -67.7) -> (-70.1621, -67.7) projected
  line L36 (-70.1621, -67.7) -> (-70.1621, -65.2) projected
  line L37 (-70.1621, -65.2) -> (-67.1621, -65.2) projected
  arc A10 (-67.1621, -65.2) -> (-64.1621, -62.2) centre (-67.1621, -62.2) ccw projected
  line L38 (-64.1621, -62.2) -> (-64.1621, -55.1072) projected
  arc A11 (-64.7971, 16.2257) -> (-64.1621, 16.7072) centre (-64.6621, 16.7072) ccw projected
  line L39 (-64.1621, 16.7072) -> (-64.1621, 23.8) projected
  arc A12 (-64.1621, 23.8) -> (-67.1621, 26.8) centre (-67.1621, 23.8) ccw projected
  line L40 (-67.1621, 26.8) -> (-70.1621, 26.8) projected
  line L41 (-70.1621, 26.8) -> (-70.1621, 29.3) projected
  line L42 (-70.1621, 29.3) -> (-59.3371, 29.3) projected
  line L43 (-59.3371, 29.3) -> (-59.3371, 30.8) projected
  line L44 (-59.3371, 30.8) -> (-78.8451, 30.8) projected
  line L45 (-78.8451, 16.3) -> (-78.8451, 30.8) projected
  line L46 (-65.3371, 16.3) -> (-78.8451, 16.3) projected
  arc A13 (-64.7971, 16.2257) -> (-65.3371, 16.3) centre (-65.3371, 14.3) ccw projected
  circle A14 centre (-67.4121, 21.8) radius 1.2295 projected
  circle A15 centre (-74.1621, 21.8) radius 1.2295 projected
hole "Hole1" at (-74.1621, -60.2, 2) at (-67.4121, -60.2, 2) at (-74.1621, 21.8, 2) at (-67.4121, 21.8, 2) at (-9.75, 13.15, 2) at (3.25, 13.15, 2) at (3.25, 6.65, 2) at (3.25, -45.05, 2) at (3.25, -51.55, 2) at (-9.75, -51.55, 2) direction (0, 0, -1) diameter 3.6 end through all clearance for "Countersunk Flat Head Screw ISO 2009/7046" size "M3" standard "ISO"
equation "\"d12\" = d11"
equation "\"d13\" = d11"
equation "\"d14\" = d11"
equation "\"d15\" = d11"
equation "\"d16\" = d11"
equation "\"d17\" = d11"
equation "\"d18\" = d11"
equation "\"d25\" = d11"
equation "\"d27\" = d11"
equation "\"d28\" = d11"
equation "\"d29\" = d11"
equation "\"d30\" = d11"
equation "\"d31\" = d11"
equation "\"d32\" = d11"
equation "\"d33\" = d11"
equation "\"d34\" = d11"
equation "\"d35\" = d11"
equation "\"d36\" = d11"
equation "\"d37\" = d11"
equation "\"d38\" = d11"
equation "\"d39\" = d11"
equation "\"d40\" = d11"
equation "\"d41\" = d11"
equation "\"d42\" = d11"
equation "\"d43\" = d11"
equation "\"d44\" = d11"
equation "\"d45\" = d11"
equation "\"d46\" = d11"
body "Solid1"
